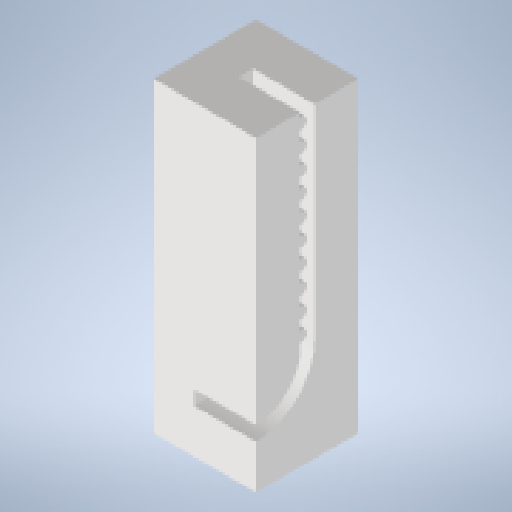
# Autodesk Inventor part: BeltClampTensioner
Saved by Autodesk Inventor 2023 (Build 270158000, 158)
## iProperties
Created: 2023-08-21
Part Number: BeltClampTensioner
Material: Generic
Document SubType Name: Modeling
Designer: Felix
Density: 1 g/cm^3
Appearance: Default
Author: Felix
Autodesk Inventor part; units mm, degrees
ref_plane "YZ Plane" through (0, 0, 0) normal (1, 0, 0) x (0, 1, 0)
ref_plane "XZ Plane" through (0, 0, 0) normal (0, 1, 0) x (-1, 0, 0)
ref_plane "XY Plane" through (0, 0, 0) normal (0, 0, 1) x (1, 0, 0)
sketch "Sketch1" plane through (0, 0, 0) normal (1, 0, 0) x (0, 1, 0)
  line L0 (0, 0) -> (-30, 0)
  line L1 (0, 0) -> (0, -4.3)
  arc A0 (-1.5, -4.5) -> (-0.5, -4.5) centre (-1, -4.5) ccw
  line L2 (-0.5, -4.5) -> (-0.5, -4.3)
  line L3 (-1.5, -4.5) -> (-1.5, -4.3)
  line L4 (0, -4.3) -> (-0.5, -4.3)
  line L5 (-1.5, -4.3) -> (-2, -4.3)
  line L6 (-2, -4.3) -> (-2.5, -4.3)
  arc A1 (-3.5, -4.5) -> (-2.5, -4.5) centre (-3, -4.5) ccw
  line L7 (-2.5, -4.5) -> (-2.5, -4.3)
  line L8 (-3.5, -4.5) -> (-3.5, -4.3)
  line L9 (-3.5, -4.3) -> (-4, -4.3)
  line L10 (-4, -4.3) -> (-4.5, -4.3)
  arc A2 (-5.5, -4.5) -> (-4.5, -4.5) centre (-5, -4.5) ccw
  line L11 (-4.5, -4.5) -> (-4.5, -4.3)
  line L12 (-5.5, -4.5) -> (-5.5, -4.3)
  line L13 (-5.5, -4.3) -> (-6, -4.3)
  line L14 (-6, -4.3) -> (-6.5, -4.3)
  arc A3 (-7.5, -4.5) -> (-6.5, -4.5) centre (-7, -4.5) ccw
  line L15 (-6.5, -4.5) -> (-6.5, -4.3)
  line L16 (-7.5, -4.5) -> (-7.5, -4.3)
  line L17 (-7.5, -4.3) -> (-8, -4.3)
  line L18 (-8, -4.3) -> (-8.5, -4.3)
  arc A4 (-9.5, -4.5) -> (-8.5, -4.5) centre (-9, -4.5) ccw
  line L19 (-8.5, -4.5) -> (-8.5, -4.3)
  line L20 (-9.5, -4.5) -> (-9.5, -4.3)
  line L21 (-9.5, -4.3) -> (-10, -4.3)
  line L22 (-10, -4.3) -> (-10.5, -4.3)
  arc A5 (-11.5, -4.5) -> (-10.5, -4.5) centre (-11, -4.5) ccw
  line L23 (-10.5, -4.5) -> (-10.5, -4.3)
  line L24 (-11.5, -4.5) -> (-11.5, -4.3)
  line L25 (-11.5, -4.3) -> (-12, -4.3)
  line L26 (-12, -4.3) -> (-12.5, -4.3)
  arc A6 (-13.5, -4.5) -> (-12.5, -4.5) centre (-13, -4.5) ccw
  line L27 (-12.5, -4.5) -> (-12.5, -4.3)
  line L28 (-13.5, -4.5) -> (-13.5, -4.3)
  line L29 (-13.5, -4.3) -> (-14, -4.3)
  line L30 (-14, -4.3) -> (-14.5, -4.3)
  arc A7 (-15.5, -4.5) -> (-14.5, -4.5) centre (-15, -4.5) ccw
  line L31 (-14.5, -4.5) -> (-14.5, -4.3)
  line L32 (-15.5, -4.5) -> (-15.5, -4.3)
  line L33 (-15.5, -4.3) -> (-16, -4.3)
  line L34 (-16, -4.3) -> (-16.5, -4.3)
  arc A8 (-17.5, -4.5) -> (-16.5, -4.5) centre (-17, -4.5) ccw
  line L35 (-16.5, -4.5) -> (-16.5, -4.3)
  line L36 (-17.5, -4.5) -> (-17.5, -4.3)
  line L37 (-17.5, -4.3) -> (-18, -4.3)
  line L38 (-18, -4.3) -> (-18.5, -4.3)
  arc A9 (-19.5, -4.5) -> (-18.5, -4.5) centre (-19, -4.5) ccw
  line L39 (-18.5, -4.5) -> (-18.5, -4.3)
  line L40 (-19.5, -4.5) -> (-19.5, -4.3)
  line L41 (-19.5, -4.3) -> (-20, -4.3)
  line L42 (-20, -4.3) -> (-20, -5.7)
  line L43 (-20, -5.7) -> (0, -5.7)
  line L44 (0, -5.7) -> (0, -10)
  line L45 (0, -10) -> (-30, -10)
  line L46 (-30, -10) -> (-30, 0)
  line L47 (-20, -5) -> (0, -5) construction
  dimension "d1" = 2
  dimension "d2" = 1
  dimension "d4" = 1
  dimension "d5" = 0.2
  dimension "d8" = 2
  dimension "d13" = 10
  dimension "d14" = 1.4
  dimension "d15" = 10
  constraints: 96 end point, 20 point on circle, 10 centre point, 10 perpendicular, 3 horizontal, 2 collinear, 2 tangent, 2 vertical, 1 midpoint, 109 other
  measures "d1" distance of L1.end L5.end
  measures "d2" diameter of A0
  measures "d4" distance from line of L1 A0.centre
  measures "d5" distance from line of L4 A0.centre
  measures "d8" distance of L1.end L6.start
  measures "d13" distance between parallel lines of L46 L42
  measures "d14" distance between parallel lines of L4 L43
  measures "d15" distance between parallel lines of L0 L45
extrude "Extrusion1" add sketch "Sketch1" along normal blind 10
sketch "Sketch2" plane through (0, -30, -10) normal (0, -1, 0) x (1, 0, 0)
  line L0 (0, 10) -> (0, 0) construction
  line L1 (0, 0) -> (10, 0) construction
  line L2 (10, 10) -> (10, 0) construction
  line L3 (0, 10) -> (10, 10) construction
  line L4 (0, 0) -> (10, 0) construction
  line L5 (0, 5.7) -> (0, 10) construction
  line L6 (10, 0) -> (0, 10) construction
  line L7 (0, 10) -> (10, 10) construction
  line L8 (10, 10) -> (0, 0) construction
  line L9 (0, 5) -> (10, 5) construction
  point P0 (5, 5)
  constraints: 4 end point, 1 midpoint
hole "Hole1" at (5, -30, -5) direction (0, 1, 0) diameter 4.3 depth 8
sketch "Sketch3" plane through (0, 0, 0) normal (-1, 0, 0) x (0, 0, 1)
  line L0 (-10, -30) -> (-10, 0) construction
  line L1 (0, 0) -> (0, -30) construction
  line L2 (0, -30) -> (-10, -30) projected
  line L3 (-4.3, 0) -> (0, 0) projected
  line L4 (-10, -30) -> (0, -30)
  line L5 (0, -30) -> (0, 0)
  line L6 (0, 0) -> (-10, 0)
  line L7 (-10, 0) -> (-10, -30)
  constraints: 8 end point, 2 parallel, 1 horizontal, 1 perpendicular
extrude "Extrusion2" add sketch "Sketch3" against normal blind 4
sketch "Sketch4" plane through (10, 0, 0) normal (1, 0, 0) x (0, 0, -1)
  line L0 (0, 0) -> (0, -30) construction
  line L1 (0, -30) -> (10, -30) construction
  line L2 (10, -30) -> (10, 0) construction
  line L3 (10, 0) -> (5.7, 0) construction
  line L4 (5.7, 0) -> (5.7, -20) construction
  line L5 (5.7, -20) -> (4.3, -20) construction
  line L6 (4.3, -20) -> (4.3, -19.5) construction
  line L7 (4.3, -19.5) -> (4.5, -19.5) construction
  arc A0 (4.5, -19.5) -> (4.5, -18.5) centre (4.5, -19) ccw construction
  line L8 (4.5, -18.5) -> (4.3, -18.5) construction
  line L9 (4.3, -18.5) -> (4.3, -17.5) construction
  line L10 (4.3, -17.5) -> (4.5, -17.5) construction
  arc A1 (4.5, -17.5) -> (4.5, -16.5) centre (4.5, -17) ccw construction
  line L11 (4.5, -16.5) -> (4.3, -16.5) construction
  line L12 (4.3, -16.5) -> (4.3, -15.5) construction
  line L13 (4.3, -15.5) -> (4.5, -15.5) construction
  arc A2 (4.5, -15.5) -> (4.5, -14.5) centre (4.5, -15) ccw construction
  line L14 (4.5, -14.5) -> (4.3, -14.5) construction
  line L15 (4.3, -14.5) -> (4.3, -13.5) construction
  line L16 (4.3, -13.5) -> (4.5, -13.5) construction
  arc A3 (4.5, -13.5) -> (4.5, -12.5) centre (4.5, -13) ccw construction
  line L17 (4.5, -12.5) -> (4.3, -12.5) construction
  line L18 (4.3, -12.5) -> (4.3, -11.5) construction
  line L19 (4.3, -11.5) -> (4.5, -11.5) construction
  arc A4 (4.5, -11.5) -> (4.5, -10.5) centre (4.5, -11) ccw construction
  line L20 (4.5, -10.5) -> (4.3, -10.5) construction
  line L21 (4.3, -10.5) -> (4.3, -9.5) construction
  line L22 (4.3, -9.5) -> (4.5, -9.5) construction
  arc A5 (4.5, -9.5) -> (4.5, -8.5) centre (4.5, -9) ccw construction
  line L23 (4.5, -8.5) -> (4.3, -8.5) construction
  line L24 (4.3, -8.5) -> (4.3, -7.5) construction
  line L25 (4.3, -7.5) -> (4.5, -7.5) construction
  arc A6 (4.5, -7.5) -> (4.5, -6.5) centre (4.5, -7) ccw construction
  line L26 (4.5, -6.5) -> (4.3, -6.5) construction
  line L27 (4.3, -6.5) -> (4.3, -5.5) construction
  line L28 (4.3, -5.5) -> (4.5, -5.5) construction
  arc A7 (4.5, -5.5) -> (4.5, -4.5) centre (4.5, -5) ccw construction
  line L29 (4.5, -4.5) -> (4.3, -4.5) construction
  line L30 (4.3, -4.5) -> (4.3, -3.5) construction
  line L31 (4.3, -3.5) -> (4.5, -3.5) construction
  arc A8 (4.5, -3.5) -> (4.5, -2.5) centre (4.5, -3) ccw construction
  line L32 (4.5, -2.5) -> (4.3, -2.5) construction
  line L33 (4.3, -2.5) -> (4.3, -1.5) construction
  line L34 (4.3, -1.5) -> (4.5, -1.5) construction
  arc A9 (4.5, -1.5) -> (4.5, -0.5) centre (4.5, -1) ccw construction
  line L35 (4.5, -0.5) -> (4.3, -0.5) construction
  line L36 (4.3, -0.5) -> (4.3, 0) construction
  line L37 (4.3, 0) -> (0, 0) construction
  arc A10 (0, -24.3) -> (4.3, -20) centre (0, -20) ccw
  line L38 (0, -24.3) -> (4.3042, -24.3) construction
  arc A11 (0, -25.7) -> (5.7, -20) centre (0, -20) ccw
  line L39 (5.7, -20) -> (4.3, -20)
  line L40 (0, -24.3) -> (0, -25.7)
  point P0 (4.3, -20)
  dimension "d27" = 1.4
  dimension "d28" = 1.4
  constraints: 6 end point, 4 point on circle, 3 point on line, 2 centre point, 2 tangent, 1 collinear, 1 horizontal, 1 line through centre, 1 parallel
  measures "d27" radial gap between concentric circles of A11 A10
  measures "d28" distance of L4.end L5.end
extrude "Extrusion3" cut sketch "Sketch4" against normal up to surface (6 mm away)
equation "\"d27\" = d28"
body "Solid1"
